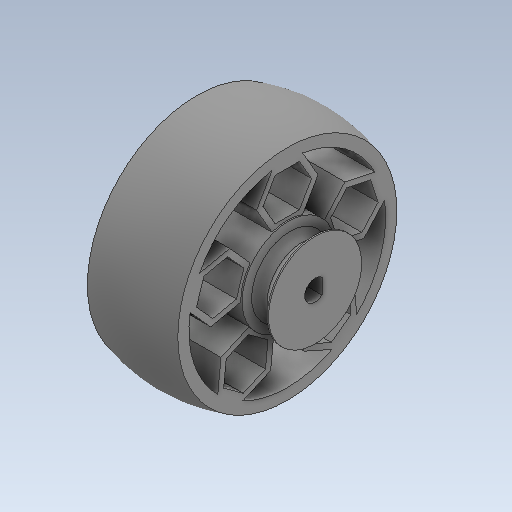
# Autodesk Inventor part: PulleyedWheelV1
Saved by Autodesk Inventor 2020 (Build 240168000, 168)
## iProperties
Created: 2023-12-21
Part Number: PulleyedWheelV1
Material: H TPU
Document SubType Name: Modeling
Designer: smz3rm
Density: 0.941117 g/cm^3
Appearance: Generic(1)
Mass: 7.24032 g
Surface Area: 71.9559 cm^2
Volume: 7.69333 cm^3
d0: 3.000 mm
d1: 1.000 mm
d3: 31.500 mm
d4: 3.000 mm
d6: 13.400 mm
d7: 4.000 mm
d8: 0.00 deg
d9: 31.500 mm
d10: 1.600 mm
d11: 0.800 mm
d16: 13.000 mm
d17: 0.00 deg
d20: 2.000 mm
d24: 1.000 mm
d26: 45.00 deg
Roundedness: 1.000 mm
BaseThickness: 3.000 mm
TopThickness: 1.778 mm
SideThickness: 4.000 mm
BodyWidth: 130.000 mm
BodyLength: 150.000 mm
BodyHeight: 30.000 mm
DriveMotorHeight: 15.000 mm
WheelDia: 33.500 mm
WheelWidth: 13.000 mm
WheelGrooveWidth: 4.000 mm
WheelGrooveDia: 13.400 mm
WheelSlotWidth: 20.000 mm
WheelPulleyDia: 2.000 mm
WheeGuardlSlotWidth: 20.000 mm
Author: smz3rm
Autodesk Inventor part; units mm, degrees
ref_plane "YZ Plane" through (0, 0, 0) normal (1, 0, 0) x (0, 1, 0)
ref_plane "XZ Plane" through (0, 0, 0) normal (0, 1, 0) x (-1, 0, 0)
ref_plane "XY Plane" through (0, 0, 0) normal (0, 0, 1) x (1, 0, 0)
sketch "Sketch1" plane through (0, 0, 0) normal (1, 0, 0) x (0, 1, 0)
  circle A0 centre (0, 0) radius 1.5
  line L0 (-25.55, 0) -> (25.55, 0) projected
  line L1 (1.118, -1) -> (-1.118, -1)
  circle A1 centre (0, 0) radius 6.7
  circle A2 centre (0, 0) radius 15.75
  circle A3 centre (0, 0) radius 12.75
  dimension "d0" = 3
  dimension "d1" = 1
  dimension "d3" = 31.5
  dimension "d4" = 3
  dimension "d6" = 13.4
  constraints: 4 centre point, 4 coincident, 2 end point, 2 point on circle, 1 horizontal
  measures "d0" diameter of A0
  measures "d1" distance between parallel lines of L0 L1
  measures "d3" diameter of A2
  measures "d4" radial gap between concentric circles of A2 A3
  measures "d6" diameter of A1
extrude "Extrusion1" add sketch "Sketch1" along normal blind 4 contours L1 A0 | A0 L0 A1 | L0 A1 A0
sketch "Sketch3" plane through (0, 0, 0) normal (0, 0, 1) x (1, 0, 0)
  line L0 (0, 6.7) -> (4, 6.7) projected
  line L1 (-0.8, 0) -> (4.8, 0) projected
  circle A0 centre (1.3858, 5.7) radius 1
  line L2 (0.4001, 5.5312) -> (0.2, 6.7)
  line L3 (0, 6.7) -> (4, 6.7) projected
  line L4 (0, 10) -> (4, 10) projected
  line L5 (0, 6.7) -> (4, 6.7) projected
  line L6 (3.8, 6.7) -> (2.0929, 4.9929)
  line L7 (3.8, 6.7) -> (3.8, 6.7)
  line L8 (3.8, 6.7) -> (4, 6.7)
  line L9 (4, -6.7) -> (4, 6.7) projected
  line L10 (4, 6.7) -> (4, 6.7)
  line L11 (0, -6.7) -> (0, 6.7) projected
  line L12 (0.2, 6.7) -> (0, 6.7)
  point P0 (0, 0)
  point P1 (1.3858, 6.7)
  point P2 (3.8, 6.7)
  dimension "d20" = 2
  dimension "d26" = 45
  dimension "d28" = 0.2
  constraints: 12 end point, 3 perpendicular, 3 tangent, 2 collinear, 2 point on circle, 2 point on line, 1 centre point, 1 vertical, 3 other
  measures "d20" diameter of A0
  measures "d26" angle of L0 L6
  measures "d28" distance of L0.end L6.start
revolve "Revolution1" cut sketch "Sketch3" angle 360 about axis through (-10, 0, 0) along (-1, 0, 0) contours L0 A0 L2 | L0 L6 A0 | A0
sketch "Sketch2" plane through (0, 0, 0) normal (-1, 0, 0) x (0, 0, 1)
  circle A0 centre (0, 0) radius 15.75
  circle A1 centre (0, 0) radius 14.15
  circle A2 centre (0, 0) radius 6.7 projected
  line L0 (-1, 1.118) -> (-1, -1.118) projected
  arc A3 (-1, -1.118) -> (-1, 1.118) centre (0, 0) ccw projected
  line L1 (2.2087, 13.9766) -> (4.4174, 10.151)
  line L2 (4.4174, 10.151) -> (2.2087, 6.3255)
  line L3 (2.2087, 6.3255) -> (-2.2087, 6.3255)
  line L4 (-2.2087, 6.3255) -> (-4.4174, 10.151)
  line L5 (-4.4174, 10.151) -> (-2.2087, 13.9766)
  line L6 (-2.2087, 13.9766) -> (2.2087, 13.9766)
  line L7 (0, -25.55) -> (0, 25.55) projected
  line L8 (-1.7468, 13.1766) -> (-3.4936, 10.151)
  line L9 (-3.4936, 10.151) -> (-1.7468, 7.1255)
  line L10 (-1.7468, 7.1255) -> (1.7468, 7.1255)
  line L11 (1.7468, 7.1255) -> (3.4936, 10.151)
  line L12 (3.4936, 10.151) -> (1.7468, 13.1766)
  line L13 (1.7468, 13.1766) -> (-1.7468, 13.1766)
  line L14 (-12.61, 6.4196) -> (-8.2892, 7.338)
  line L15 (-13.975, 2.2184) -> (-12.61, 6.4196)
  line L16 (-11.0192, -1.0643) -> (-13.975, 2.2184)
  line L17 (-6.6984, -0.1459) -> (-11.0192, -1.0643)
  line L18 (-10.7338, -0.1858) -> (-7.3165, 0.5406)
  line L19 (-7.3165, 0.5406) -> (-6.2369, 3.8632)
  line L20 (-6.2369, 3.8632) -> (-8.5746, 6.4594)
  line L21 (-8.2892, 7.338) -> (-5.3334, 4.0553)
  line L22 (-5.3334, 4.0553) -> (-6.6984, -0.1459)
  line L23 (-8.5746, 6.4594) -> (-11.9919, 5.7331)
  line L24 (-11.9919, 5.7331) -> (-13.0714, 2.4105)
  line L25 (-13.0714, 2.4105) -> (-10.7338, -0.1858)
  line L26 (-10.0021, -10.009) -> (-9.5403, -5.6159)
  line L27 (-6.4284, -12.6055) -> (-10.0021, -10.009)
  line L28 (-2.3929, -10.8088) -> (-6.4284, -12.6055)
  line L29 (-1.9312, -6.4157) -> (-2.3929, -10.8088)
  line L30 (-3.1402, -10.2658) -> (-2.7751, -6.7914)
  line L31 (-2.7751, -6.7914) -> (-5.6014, -4.7379)
  line L32 (-5.6014, -4.7379) -> (-8.793, -6.1589)
  line L33 (-9.5403, -5.6159) -> (-5.5049, -3.8192)
  line L34 (-5.5049, -3.8192) -> (-1.9312, -6.4157)
  line L35 (-8.793, -6.1589) -> (-9.1582, -9.6333)
  line L36 (-9.1582, -9.6333) -> (-6.3318, -11.6868)
  line L37 (-6.3318, -11.6868) -> (-3.1402, -10.2658)
  line L38 (6.4284, -12.6055) -> (2.3929, -10.8088)
  line L39 (10.0021, -10.009) -> (6.4284, -12.6055)
  line L40 (9.5403, -5.6159) -> (10.0021, -10.009)
  line L41 (5.5049, -3.8192) -> (9.5403, -5.6159)
  line L42 (8.793, -6.1589) -> (5.6014, -4.7379)
  line L43 (5.6014, -4.7379) -> (2.7751, -6.7914)
  line L44 (2.7751, -6.7914) -> (3.1402, -10.2658)
  line L45 (2.3929, -10.8088) -> (1.9312, -6.4157)
  line L46 (1.9312, -6.4157) -> (5.5049, -3.8192)
  line L47 (3.1402, -10.2658) -> (6.3318, -11.6868)
  line L48 (6.3318, -11.6868) -> (9.1582, -9.6333)
  line L49 (9.1582, -9.6333) -> (8.793, -6.1589)
  line L50 (13.975, 2.2184) -> (11.0192, -1.0643)
  line L51 (12.61, 6.4196) -> (13.975, 2.2184)
  line L52 (8.2892, 7.338) -> (12.61, 6.4196)
  line L53 (5.3334, 4.0553) -> (8.2892, 7.338)
  line L54 (8.5746, 6.4594) -> (6.2369, 3.8632)
  line L55 (6.2369, 3.8632) -> (7.3165, 0.5406)
  line L56 (7.3165, 0.5406) -> (10.7338, -0.1858)
  line L57 (11.0192, -1.0643) -> (6.6984, -0.1459)
  line L58 (6.6984, -0.1459) -> (5.3334, 4.0553)
  line L59 (10.7338, -0.1858) -> (13.0714, 2.4105)
  line L60 (13.0714, 2.4105) -> (11.9919, 5.7331)
  line L61 (11.9919, 5.7331) -> (8.5746, 6.4594)
  point P0 (0, 10.151)
  point P1 (2.2087, 6.3255)
  point P2 (-12.61, 6.4196)
  point P3 (-5.3334, 4.0553)
  point P4 (-13.975, 2.2184)
  point P5 (-6.6984, -0.1459)
  point P6 (-5.5049, -3.8192)
  point P7 (-6.4284, -12.6055)
  point P8 (-1.9312, -6.4157)
  point P9 (1.9312, -6.4157)
  point P10 (6.4284, -12.6055)
  point P11 (10.0021, -10.009)
  point P12 (5.5049, -3.8192)
  point P13 (6.6984, -0.1459)
  point P14 (13.975, 2.2184)
  point P15 (12.61, 6.4196)
  point P16 (5.3334, 4.0553)
  dimension "d9" = 31.5
  dimension "d10" = 1.6
  dimension "d11" = 0.8
  dimension "d31" = 360
  constraints: 120 end point, 2 centre point, 2 coincident, 2 point on circle, 1 point on line, 141 other
  measures "d9" diameter of A0
  measures "d10" radial gap between concentric circles of A0 A1
  measures "d11" distance between parallel lines of L5 L8
extrude "Extrusion2" add sketch "Sketch2" along normal blind 13 contours A0 L7 A1 | L7 A1 A0 | L7 L6 A1 | A1 L6 L7 | L1 L2 A2 L7 L10 L11 L12 L13 L6 | L6 L7 L13 L8 L9 L10 A2 L4 L5 | A1 L27 | L27 L26 L33 A2 L29 L28 | L39 A1 | L38 L45 A2 L41 L40 L39 | L7 A3 L3 A2 L58 L46 | A2 L34 L22 L3 L7 A3 L0 | A1 L51 | L51 L50 L57 A2 L53 L52 | L15 A1 | L14 L21 A2 L17 L16 L15 | A2 L34 | L46 A2 | L7 A3 | A3 L0 L7 | L3 L7 A2 | A2 L7 L3 | A2 L58 | L22 A2
sketch "Sketch4" plane through (0, 0, 0) normal (0, 0, 1) x (1, 0, 0)
  line L0 (0, 15.75) -> (-13, 15.75) projected
  line L1 (-13, 15.75) -> (-13, -15.75) projected
  arc A0 (0, 15.75) -> (-13, 15.75) centre (-6.5, -4.875) ccw
  line L2 (-15.6, 0) -> (2.6, 0) projected
  point P0 (0, 0)
  point P1 (-6.5, 16.75)
  dimension "d24" = 1
  constraints: 3 point on circle, 1 centre point
  measures "d24" distance from line of L0 point (-6.5, 16.75)
revolve "Revolution2" add sketch "Sketch4" angle 360 about axis through (-10, 0, 0) along (1, 0, 0)
equation "\"d6\" = WheelGrooveDia"
equation "\"d7\" = WheelGrooveWidth"
equation "\"d20\" = WheelPulleyDia"
equation "\"d9\" = WheelDia - 2 * Roundedness"
equation "\"d16\" = WheelWidth"
equation "\"d24\" = Roundedness"
equation "\"Roundedness\" = 1"
equation "\"WheelGrooveDia\" = 13.4"
equation "\"WheelGrooveWidth\" = 4"
equation "\"WheelPulleyDia\" = 2"
equation "\"WheelDia\" = 33.5"
equation "\"WheelWidth\" = 13"
body "Solid1"
